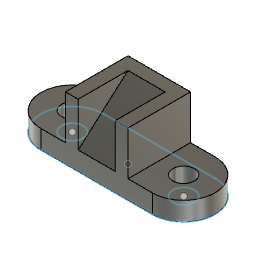
A2 (Autodesk Fusion 360 design; units mm, degrees)
Autodesk Fusion 360 part; units mm, degrees
sketch "Sketch1" plane through (0, 0, 0) normal (0, 0, 1) x (1, 0, 0)
  line L0 (57, 32) -> (-57, 32)
  line L1 (-57, -32) -> (57, -32)
  circle A0 centre (57, 0) radius 11
  circle A1 centre (-57, 0) radius 11
  arc A2 (-57, 32) -> (-57, -32) centre (-57, 0) ccw
  arc A3 (57, -32) -> (57, 32) centre (57, 0) ccw
  dimension "d1" = 114
  dimension "d2" = 64
  dimension "d5" = 22
  dimension "d6" = 22
  constraint horizontal L0
  constraint parallel L0 L1
  constraint concentric A0 A3
  constraint concentric A1 A2
  measures "d1" distance of L1.start L1.end
  measures "d2" distance of L0.end L1.start
  measures "d5" diameter of A0
  measures "d6" diameter of A1
extrude "Extrude1" add sketch "Sketch1" along normal blind 19
sketch "Sketch2" plane through (0, 0, 19) normal (0, 0, 1) x (-1, 0, 0)
  circle A0 centre (-57, 0) radius 11
  circle A1 centre (57, 0) radius 11
  arc A2 (-57, 32) -> (-57, -32) centre (-57, 0) ccw
  line L0 (-57, -32) -> (57, -32)
  arc A3 (57, -32) -> (57, 32) centre (57, 0) ccw
  line L1 (57, 32) -> (-57, 32)
  line L2 (32, -32) -> (-32, -32)
  line L3 (-32, -32) -> (-32, 32)
  line L4 (-32, 32) -> (32, 32)
  line L5 (32, 32) -> (32, -32)
  line L6 (0, -32) -> (0, 32) construction
  line L7 (19, 32) -> (-19, 32)
  line L8 (-19, 32) -> (-19, -19)
  line L9 (-19, -19) -> (19, -19)
  line L10 (19, -19) -> (19, 32)
  dimension "d9" = 64
  dimension "d10" = 64
  dimension "d11" = 32
  dimension "d12" = 38
  dimension "d13" = 51
  dimension "d14" = 19
  constraint horizontal L2
  constraint vertical L3
  constraint horizontal L4
  constraint vertical L5
  constraint coincident L0 L2.start
  constraint midpoint L0 L6.start
  constraint midpoint L1 L6.end
  constraint horizontal L7
  constraint vertical L8
  constraint horizontal L9
  constraint vertical L10
  constraint coincident L1 L7.start
  measures "d9" distance of L2.start L2.end
  measures "d10" distance of L2.start L4.end
  measures "d11" distance of L5 L6
  measures "d12" distance of L7.start L7.end
  measures "d13" distance of L7.start L9.end
  measures "d14" distance of L6 L8
extrude "Extrude2" add sketch "Sketch2" along normal blind 45 contours L0 L1 L2 L3 L4 L5 L8 L9 L10
sketch "Sketch3" plane through (0, 0, 0) normal (1, 0, 0) x (0, 1, 0)
  line L0 (-32, 19) -> (19, 19)
  line L1 (19, 19) -> (19, 64)
  line L2 (19, 64) -> (-32, 19)
  dimension "d17" = 51
  constraint horizontal L0
  constraint perpendicular L0 L1
  measures "d17" distance of L0.start L0.end
extrude "Extrude3" add sketch "Sketch3" along normal mid plane 38
equation "d15 = 64 mm - 19 mm"
named bodies: "A2"
